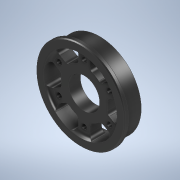
# Autodesk Inventor part: 3inWheelHalf
Saved by Autodesk Inventor 2020 (Build 240168000, 168)
## iProperties
Created: 2019-07-10
Part Number: 3inWheelHalf
Material: ABS Plastic
Document SubType Name: Modeling
Designer: Connor
Density: 1.06 g/cm^3
Appearance: Glossy - Black
Author: Connor
Autodesk Inventor part; units mm, degrees
ref_plane "YZ Plane" through (0, 0, 0) normal (1, 0, 0) x (0, 1, 0)
ref_plane "XZ Plane" through (0, 0, 0) normal (0, 1, 0) x (-1, 0, 0)
ref_plane "XY Plane" through (0, 0, 0) normal (0, 0, 1) x (1, 0, 0)
sketch "Sketch1" plane through (0, 0, 0) normal (0, 1, 0) x (-1, 0, 0)
  line L0 (0, 0) -> (-30.1625, 0)
  line L1 (-30.1625, 0) -> (-30.1625, 3.175)
  line L2 (-30.1625, 3.175) -> (-36.5125, 3.175)
  line L3 (-36.5125, 3.175) -> (-36.5125, 0)
  line L4 (-36.5125, 0) -> (-34.1122, 0)
  line L5 (-34.1122, 0) -> (-34.1122, -12.7)
  line L6 (-34.1122, -12.7) -> (-30.1625, -12.7)
  line L7 (-30.1625, -12.7) -> (-30.1625, -9.525)
  line L8 (-30.1625, -9.525) -> (0, -9.525)
  line L9 (0, -9.525) -> (0, 0)
  dimension "d0" = 36.5125
  dimension "d1" = 6.35
  dimension "d2" = 34.1122
  dimension "d3" = 3.175
  dimension "d12" = 12.7
  dimension "d13" = 3.175
  constraints: 20 end point, 8 perpendicular, 2 point on line, 1 collinear, 1 horizontal
  measures "d0" distance between parallel lines of L9 L3
  measures "d1" distance of L1.end L2.end
  measures "d2" distance between parallel lines of L5 L9
  measures "d3" distance of L2.end L3.end
  measures "d12" distance between parallel lines of L4 L6
  measures "d13" distance between parallel lines of L6 L8
revolve "Revolution1" add sketch "Sketch1" angle 360 about axis through (0, 0, -9.525) along (0, 0, 1)
sketch "Sketch2" plane through (0, 0, 0) normal (0, 0, 1) x (1, 0, 0)
  circle A0 centre (0, 0) radius 12.7
  circle A1 centre (0, 0) radius 19.05
  circle A2 centre (0, 0) radius 30.1625
  line L0 (0, 0) -> (0, 30.1625) construction
  line L1 (0, 0) -> (26.121491, 15.08125) construction
  circle A3 centre (0, 0) radius 30.1625 construction
  line L2 (4.7625, 29.78414) -> (4.7625, 18.445083)
  line L3 (13.592661, 13.346988) -> (23.412572, 19.016516)
  dimension "d5" = 25.4
  dimension "d6" = 38.1
  dimension "d7" = 60
  dimension "d8" = 4.7625
  dimension "d9" = 4.7625
  constraints: 8 end point, 5 point on circle, 2 centre point, 2 coincident, 2 vertical, 1 parallel, 2 other
  measures "d5" diameter of A0
  measures "d6" diameter of A1
  measures "d7" angle of L1 L0
  measures "d8" distance between parallel lines of L2 L0
  measures "d9" distance between parallel lines of L1 L3
extrude "Extrusion1" cut sketch "Sketch2" against normal through all contours A0 | A1 L2 A2 L3 picked at (13.637832, 22.476088)
pattern_circular "Circular Pattern1" count 6 over 360 about axis through (0, 0, 0) along (0, 0, -1) of "Extrusion1"
fillet "Fillet1" radius 3.175 30 edges at (-18.3552, -5.0981, -4.7625) (-18.3552, 5.0981, -4.7625) (13.5927, -13.347, -4.7625) (4.7625, -18.4451, -4.7625) (18.3552, 5.0981, -4.7625) (18.3552, -5.0981, -4.7625) (-4.7625, -18.4451, -4.7625) (-13.5927, -13.347, -4.7625) (-13.5927, 13.347, -4.7625) (-4.7625, 18.4451, -4.7625) (4.7625, 18.4451, -4.7625) (13.5927, 13.347, -4.7625) (-4.7625, 29.7841, -4.7625) (-23.4126, 19.0165, -4.7625) (-28.1751, 10.7676, -4.7625) (-28.1751, -10.7676, -4.7625) (-23.4126, -19.0165, -4.7625) (4.7625, -29.7841, -4.7625) (-4.7625, -29.7841, -4.7625) (23.4126, -19.0165, -4.7625) (28.1751, -10.7676, -4.7625) (23.4126, 19.0165, -4.7625) (28.1751, 10.7676, -4.7625) (4.7625, 29.7841, -4.7625) (-26.1215, 15.0812, 0) (0, 30.1625, 0) (26.1215, 15.0813, 0) (26.1215, -15.0812, 0) (0, -30.1625, 0) (-26.1215, -15.0813, 0)
sketch "Sketch3" plane through (0, 0, 0) normal (0, 0, 1) x (-0.5, 0.8660254, 0)
  circle A0 centre (0, 0) radius 23.8125 construction
  point P0 (0, 0)
  point P1 (0, 23.8125)
  point P2 (-20.62223, 11.90625)
  point P3 (-20.62223, -11.90625)
  point P4 (0, -23.8125)
  point P5 (20.62223, -11.90625)
  point P6 (20.62223, 11.90625)
  dimension "d18" = 47.625
  dimension "d21" = 360
  constraints: 2 vertical alignment, 1 coincident, 9 other
hole "Hole1" at (-20.62223, -11.90625, 0) at (0, -23.8125, 0) at (20.62223, -11.90625, 0) at (20.62223, 11.90625, 0) at (0, 23.8125, 0) at (-20.62223, 11.90625, 0) direction (0, 0, -1) diameter 4.318 end through all
chamfer "Chamfer1" distance 0.79375 angle 45 1 edges at (-36.5125, 0, 3.175)
body "Solid1"
